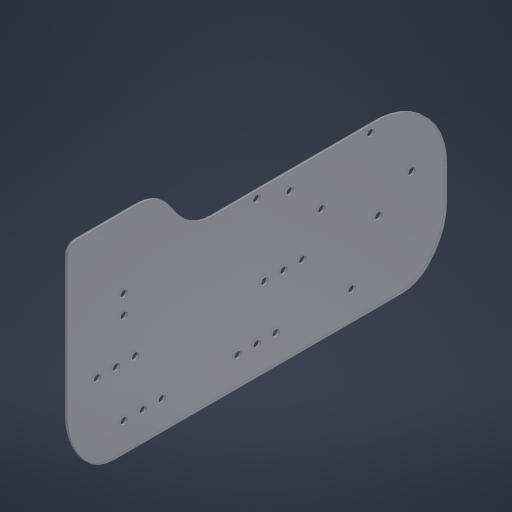
# Autodesk Inventor part: dtplate
Saved by Autodesk Inventor 2024 (Build 280153000, 153)
## iProperties
Created: 2023-11-04
Part Number: dtplate
Material: Generic
Document SubType Name: Modeling
Designer: macbook
Density: 1 g/cm^3
Appearance: Clear - Light
Author: macbook
Autodesk Inventor part; units mm, degrees
ref_plane "YZ Plane" through (0, 0, 0) normal (1, 0, 0) x (0, 1, 0)
ref_plane "XZ Plane" through (0, 0, 0) normal (0, 1, 0) x (-1, 0, 0)
ref_plane "XY Plane" through (0, 0, 0) normal (0, 0, 1) x (1, 0, 0)
sketch "Sketch1" plane through (0, 0, 0) normal (1, 0, 0) x (0, 1, 0)
  line L0 (-0.0645, -0.0614) -> (-0.0645, 12.6386) construction
  line L1 (-0.0645, 12.6386) -> (-0.0645, 25.3386) construction
  line L2 (-0.0645, -0.0614) -> (33.5905, -0.0614) construction
  line L3 (-0.0645, -0.0614) -> (33.5814, 17.8149) construction
  line L4 (33.5814, 17.8149) -> (33.5814, 30.5149) construction
  line L5 (33.5814, 30.5149) -> (33.5814, 43.2149) construction
  line L6 (-0.0645, -0.0614) -> (-0.0645, -25.4614) construction
  line L7 (-0.0645, -25.4614) -> (-0.0645, -50.8614) construction
  line L8 (-0.0645, -50.8614) -> (-0.0645, -88.9614) construction
  line L9 (-0.0645, -88.9614) -> (-0.0645, -127.0614) construction
  line L10 (-0.0645, -127.0614) -> (33.5905, -127.0614) construction
  line L11 (-0.0645, -127.0614) -> (33.5905, -144.9206) construction
  line L12 (-0.0645, -50.8614) -> (33.5905, -50.8614) construction
  line L13 (-0.0645, -50.8614) -> (33.5905, -68.7206) construction
  line L14 (33.5905, -68.7206) -> (33.5905, -81.4206) construction
  line L15 (33.5905, -81.4206) -> (33.5905, -94.1206) construction
  line L16 (33.5905, -144.9206) -> (33.5905, -106.8206) construction
  line L17 (33.5905, -106.8206) -> (96.5027, -106.8206) construction
  line L18 (33.5905, -144.9206) -> (56.4857, -106.8206) construction
  line L19 (33.5905, -68.7206) -> (56.4857, -106.8206) construction
  line L20 (-0.0645, -50.8614) -> (-0.0645, -63.5614) construction
  line L21 (-0.0645, -63.5614) -> (-0.0645, -76.2614) construction
  line L22 (33.5905, -0.0614) -> (67.2455, -0.0614) construction
  line L23 (67.2455, -0.0614) -> (33.5814, 17.8149) construction
  line L24 (67.2455, -0.0614) -> (67.2455, 25.3386) construction
  line L25 (67.2455, 25.3386) -> (67.2455, 25.3386) construction
  line L26 (67.2455, 25.3386) -> (73.5955, 25.3386) construction
  line L27 (67.2455, 25.3386) -> (60.8955, 25.3386) construction
  line L28 (-19.1145, -0.0711) -> (-19.1145, -127.0711)
  line L29 (-19.1145, -0.0711) -> (-19.1145, 32.0046)
  line L30 (-19.1145, 63.4289) -> (18.9855, 63.4289) construction
  line L31 (39.9379, -190.511) -> (19.05, -190.5323)
  line L32 (-19.05, -190.571) -> (-19.0726, -168.346) construction
  line L33 (-19.1145, 63.4289) -> (18.9855, 63.4289)
  line L34 (-19.1145, 63.4289) -> (-19.1145, 41.2039) construction
  line L35 (-19.05, -190.571) -> (-19.0726, -168.346)
  line L36 (-19.05, -190.571) -> (19.05, -190.5323) construction
  arc A0 (-11.2228, -178.4175) -> (19.05, -190.5323) centre (19.0055, -146.7627) ccw
  arc A1 (18.9855, 63.4289) -> (-10.4946, 51.0726) centre (22.5956, 13.4704) ccw
  line L37 (-19.1145, 41.2039) -> (-19.1145, 63.4289)
  line L38 (-19.081, -160.0737) -> (-19.1145, -127.0711)
  line L39 (19.05, -190.5323) -> (-19.05, -190.571)
  arc A2 (-10.4946, 51.0726) -> (-19.1145, 32.0046) centre (6.2855, 32.0046) ccw
  arc A3 (-19.081, -160.0737) -> (-11.2228, -178.4175) centre (6.319, -160.0479) ccw
  line L40 (82.55, -43.1133) -> (82.55, -47.5335)
  line L41 (82.55, -190.4677) -> (82.55, -154.3842)
  line L42 (82.55, 3.175) -> (82.55, 63.4289)
  line L43 (82.55, 63.4289) -> (18.9855, 63.4289)
  line L44 (19.05, -190.5323) -> (50.8, -190.5)
  line L45 (82.55, -190.4677) -> (82.55, -117.4427)
  arc A4 (59.4372, -181.357) -> (82.55, -117.4427) centre (-17.378, -117.4427) ccw
  arc A5 (39.9379, -190.511) -> (59.4372, -181.357) centre (39.9121, -165.1111) ccw
  line L46 (82.55, 63.4289) -> (82.55, -38.1711)
  line L47 (82.55, 63.4289) -> (114.3, 63.4289)
  line L48 (120.65, 57.0789) -> (120.65, 15.7647)
  arc A6 (108.6074, -5.8395) -> (95.5578, -16.5987) centre (141.4695, -58.9906) ccw
  arc A7 (84.9949, -32.2402) -> (82.55, -43.1133) centre (107.95, -43.1133) ccw
  arc A8 (108.6074, -5.8395) -> (120.65, 15.7647) centre (95.25, 15.7647) ccw
  arc A9 (120.65, 57.0789) -> (114.3, 63.4289) centre (114.3, 57.0789) ccw
  line L49 (82.55, -190.4677) -> (82.55, -79.4019)
  line L50 (82.55, -63.4677) -> (84.1375, -63.4677)
  line L51 (82.55, -117.4427) -> (82.55, -134.9348)
  line L52 (33.5905, -144.9206) -> (33.5905, -167.1456)
  line L53 (33.5905, -167.1456) -> (48.1955, -167.1456)
  line L54 (82.55, -117.4427) -> (82.55, -113.6327)
  line L55 (82.55, -63.4677) -> (88.9, -63.4677)
  line L56 (82.55, -63.4677) -> (82.55, -76.1677)
  line L57 (82.55, -63.4677) -> (82.55, -50.7677)
  arc A10 (88.9, -63.4677) -> (84.7021, -52.298) centre (76.3064, -61.827) ccw
  arc A11 (82.55, -47.5335) -> (84.7021, -52.298) centre (88.9, -47.5335) ccw
  arc A12 (84.7021, -74.6374) -> (82.55, -79.4019) centre (88.9, -79.4019) ccw
  line L58 (82.55, -63.4677) -> (84.1375, -63.4677)
  line L59 (84.1375, -63.4677) -> (84.1375, -139.6677)
  line L60 (82.55, -117.4427) -> (95.25, -139.6677)
  line L61 (95.25, -139.6677) -> (75.6405, -153.9552)
  line L62 (82.55, -63.4677) -> (77.47, -63.4677)
  line L63 (77.47, -63.4677) -> (77.47, -85.6927)
  line L64 (88.9, -63.4677) -> (88.9, -139.6677)
  arc A13 (39.9379, -190.511) -> (88.9, -139.6677) centre (41.7296, -143.2396) ccw
  line L65 (88.9, -63.4677) -> (88.8195, -33.8988)
  arc A14 (95.5578, -16.5987) -> (88.8195, -33.8988) centre (114.2194, -33.8296) ccw
  point P0 (82.55, -106.8206)
  point P1 (120.65, 63.4289)
  point P2 (120.65, -0.0711)
  point P3 (82.55, -148.9209)
  point P4 (43.6175, -190.5073)
  point P5 (88.7962, -25.3679)
  point P6 (82.55, -167.1456)
  point P7 (88.8909, -60.1177)
  dimension "d81" = 33.655
  dimension "d82" = 38.1
  dimension "d86" = 12.7
  dimension "d93" = 25.4
  dimension "d94" = 38.1
  dimension "d95" = 38.1
  dimension "d98" = 33.655
  dimension "d109" = 38.1
  dimension "d110" = 12.7
  dimension "d111" = 12.7
  dimension "d112" = 38.1
  dimension "d113" = 44.45
  dimension "d114" = 12.7
  dimension "d115" = 12.7
  dimension "d116" = 33.655
  dimension "d117" = 25.4
  dimension "d118" = 0
  dimension "d119" = 6.35
  dimension "d120" = 6.35
  dimension "d122" = 19.05
  dimension "d126" = 127
  dimension "d127" = 63.5
  dimension "d129" = 38.1
  dimension "d130" = 22.225
  dimension "d131" = 22.225
  dimension "d132" = 38.1
  dimension "d133" = 50.0888
  dimension "d134" = 25.4
  dimension "d135" = 25.4
  dimension "d137" = 31.75
  dimension "d138" = 73.025
  dimension "d139" = 25.4
  dimension "d140" = 101.6
  dimension "d141" = 38.1
  dimension "d142" = 25.4
  dimension "d143" = 6.35
  dimension "d144" = 62.4897
  dimension "d145" = 127
  dimension "d148" = 22.225
  dimension "d149" = 14.605
  dimension "d153" = 6.35
  dimension "d154" = 12.7
  dimension "d155" = 12.7
  dimension "d157" = 12.7
  dimension "d158" = 6.35
  dimension "d159" = 1.5875
  dimension "d160" = 76.2
  dimension "d161" = 5.08
  dimension "d162" = 22.225
  dimension "d163" = 38.1
  dimension "d164" = 25.4
  constraints: 132 end point, 39 point on circle, 29 point on line, 21 coincident, 19 tangent, 15 centre point, 15 vertical, 12 perpendicular, 7 horizontal, 2 equal radius, 2 parallel, 1 midpoint
  measures "d81" distance of L0.start L2.end
  measures "d82" distance of L0.start L3.end
  measures "d86" distance of L3.end L4.end
  measures "d93" distance of L6.end L7.end
  measures "d94" distance of L7.end L8.end
  measures "d95" distance of L8.end L9.end
  measures "d98" distance of L10.start L10.end
  measures "d109" distance of L12.start L13.end
  measures "d110" distance of L14.start L14.end
  measures "d111" distance of L14.end L15.end
  measures "d112" distance of L16.start L16.end
  measures "d113" distance of L16.start L18.end
  measures "d114" distance of L12.start L20.end
  measures "d115" distance of L20.end L21.end
  measures "d116" distance of L2.end L22.end
  measures "d117" distance of L22.end L24.end
  measures "d118" distance of L24.end L25.end
  measures "d119" distance of L25.end L26.end
  measures "d120" distance of L25.end L27.end
  measures "d122" distance of L0.start L28.start
  measures "d126" distance of L28.start L28.end
  measures "d127" distance of L28.start L30.start
  measures "d129" distance of L30.start L30.end
  measures "d130" distance of L30.start L34.end
  measures "d131" distance of L32.start L32.end
  measures "d132" distance of L32.start L31.end
  measures "d133" radius of A1
  measures "d134" radius of A2
  measures "d135" radius of A3
  measures "d137" distance of L31.end L44.end
  measures "d138" distance of L41.start L45.end
  measures "d139" radius of A5
  measures "d140" distance of L42.end L46.end
  measures "d141" distance of L42.end point (120.65, 63.429)
  measures "d142" radius of A7
  measures "d143" radius of A9
  measures "d144" radius of A6
  measures "d145" distance of L41.start L50.start
  measures "d148" distance of L16.start L52.end
  measures "d149" distance of L52.end L53.end
  measures "d153" distance of L50.start L55.end
  measures "d154" distance of L50.start L56.end
  measures "d155" distance of L50.start L57.end
  measures "d157" radius of A10
  measures "d158" radius of A11
  measures "d159" distance of L50.start L58.end
  measures "d160" distance of L59.start L59.end
  measures "d161" distance of L50.start L62.end
  measures "d162" distance of L62.end L63.end
  measures "d163" distance of L55.end point (88.796, -25.368)
  measures "d164" radius of A14
extrude "Extrusion1" add sketch "Sketch1" along normal blind 1.5875 contours L29 A2 A1 L43 L47 A9 L48 A8 A6 A14 L65 L55 L59 A12 L49 A4 A5 L31 A0 A3 L38 L28 | A5 A4 L61 L45 L41 A13 L44 | L44 A13 | L41 L45 L61 A13 | A4 L45 L61 | L61 L45 L60 L64 A13 | L49 A12 L59 L60 | L59 L55 L64 L60 | L65 A10
hole "Hole4" at (0, -0.0645, -0.0614) at (0, -0.0645, 12.6386) at (0, -0.0645, 25.3386) at (0, -0.0645, -127.0614) at (0, 33.5905, -144.9206) at (0, -0.0645, -50.8614) at (0, 33.5814, 43.2149) at (0, 33.5814, 30.5149) at (0, 33.5814, 17.8149) at (0, 33.5905, -68.7206) at (0, 33.5905, -81.4206) at (0, 33.5905, -94.1206) at (0, -0.0645, -63.5614) at (0, -0.0645, -76.2614) at (0, 56.4857, -106.8206) at (0, 60.8955, 25.3386) at (0, 73.5955, 25.3386) at (0, 48.1955, -167.1456) at (0, 84.1375, -63.4677) at (0, 77.47, -85.6927) at (0, 84.1375, -139.6677) direction (1, 0, 0) diameter 4.7625 end through all
body "Solid1"
